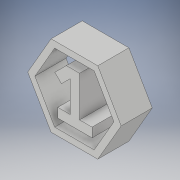
# Autodesk Inventor part: 1
Saved by Autodesk Inventor 2019 (Build 230136000, 136)
## iProperties
Created: 2018-07-31
Part Number: 1
Material: Generic
Document SubType Name: Modeling
Designer: Ge Shi
Density: 1 g/cm^3
Appearance: Default
Author: Ge Shi
Autodesk Inventor part; units mm, degrees
ref_plane "YZ Plane" through (0, 0, 0) normal (1, 0, 0) x (0, 1, 0)
ref_plane "XZ Plane" through (0, 0, 0) normal (0, 1, 0) x (-1, 0, 0)
ref_plane "XY Plane" through (0, 0, 0) normal (0, 0, 1) x (1, 0, 0)
sketch "Sketch1" plane through (0, 0, 0) normal (0, 0, 1) x (1, 0, 0)
  circle A0 centre (0, 0) radius 7.5
  line L0 (-3.75, 6.4952) -> (3.75, 6.4952)
  line L1 (3.75, 6.4952) -> (7.5, 0)
  line L2 (7.5, 0) -> (3.75, -6.4952)
  line L3 (3.75, -6.4952) -> (-3.75, -6.4952)
  line L4 (-3.75, -6.4952) -> (-7.5, 0)
  line L5 (-7.5, 0) -> (-3.75, 6.4952)
  line L6 (-3.1726, 5.4952) -> (3.1726, 5.4952)
  line L7 (3.1726, 5.4952) -> (6.3453, 0)
  line L8 (6.3453, 0) -> (3.1726, -5.4952)
  line L9 (3.1726, -5.4952) -> (-3.1726, -5.4952)
  line L10 (-3.1726, -5.4952) -> (-6.3453, 0)
  line L11 (-6.3453, 0) -> (-3.1726, 5.4952)
  line L12 (-1.294, 3.9952) -> (-3.1475, 2.1416)
  line L13 (-3.1475, 2.1416) -> (-2.0869, 1.081)
  line L14 (-2.0869, 1.081) -> (-0.6726, 2.4952)
  line L15 (-0.6726, 2.4952) -> (-0.6726, -2.4952)
  line L16 (-0.6726, -2.4952) -> (-2.6726, -2.4952)
  line L17 (-2.6726, -2.4952) -> (-2.6726, -3.9952)
  line L18 (-2.6726, -3.9952) -> (2.8274, -3.9952)
  line L19 (2.8274, -3.9952) -> (2.8274, -2.4952)
  line L20 (2.8274, -2.4952) -> (0.8274, -2.4952)
  line L21 (0.8274, -2.4952) -> (0.8274, 3.9952)
  line L22 (0.8274, 3.9952) -> (-1.294, 3.9952)
  dimension "d0" = 15
  dimension "d1" = 1
  dimension "d2" = 1.5
  dimension "d3" = 1.5
  dimension "d4" = 1.5
  dimension "d5" = 1.5
  dimension "d6" = 2
  dimension "d7" = 2
  dimension "d8" = 2
  dimension "d9" = 1.5
  dimension "d10" = 1.5
  dimension "d11" = 0.5
  dimension "d12" = 45
  constraints: 46 end point, 8 perpendicular, 3 coincident, 2 horizontal, 2 point on line, 1 vertical, 29 other
  measures "d1" distance between parallel lines of L0 L6
  measures "d2" distance between parallel lines of L21 L15
  measures "d3" distance between parallel lines of L12 L14
  measures "d4" distance from line of L22 L14.end
  measures "d5" distance between parallel lines of L18 L16
  measures "d6" distance between parallel lines of L15 L17
  measures "d7" distance between parallel lines of L19 L21
  measures "d8" distance from line of L14.end L13
  measures "d9" distance between parallel lines of L6 L22
  measures "d10" distance between parallel lines of L9 L18
  measures "d11" distance from line of L9.end L17
  measures "d12" angle of L15 L14
extrude "Extrusion1" add sketch "Sketch1" along normal blind 5 contours L2 L3 L4 L5 L0 L1 | L22 L21 L20 L19 L18 L17 L16 L15 L14 L13 L12
body "Solid1"
